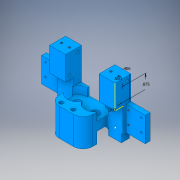
# Autodesk Inventor part: GripperBlock
Saved by Autodesk Inventor 2019 (Build 230136000, 136)
## iProperties
Created: 2019-10-02
Part Number: GripperBlock
Material: Generic
Document SubType Name: Modeling
Designer: james
Density: 1 g/cm^3
Appearance: Default(2)
Author: james
Autodesk Inventor part; units mm, degrees
ref_plane "YZ Plane" through (0, 0, 0) normal (1, 0, 0) x (0, 1, 0)
ref_plane "XZ Plane" through (0, 0, 0) normal (0, 1, 0) x (-1, 0, 0)
ref_plane "XY Plane" through (0, 0, 0) normal (0, 0, 1) x (1, 0, 0)
sketch "Sketch1" plane through (0, 0, 0) normal (1, 0, 0) x (0, 1, 0)
  line L0 (11.2985, 26.2091) -> (-33.1515, 26.2091)
  line L1 (-33.1515, 26.2091) -> (-33.1515, -24.5909)
  line L2 (-33.1515, -24.5909) -> (11.2985, -24.5909)
  line L3 (11.2985, -24.5909) -> (11.2985, 26.2091)
  point P0 (0, 0)
  dimension "d0" = 50.8
  dimension "d1" = 44.45
  constraints: 8 end point, 2 parallel, 1 horizontal, 1 perpendicular
  measures "d0" distance of L2.end L0.start
  measures "d1" distance of L0.start L0.end
extrude "Extrusion1" add sketch "Sketch1" along normal blind 165.1
sketch "Sketch2" plane through (0, 11.2985, 26.2091) normal (0, 1, 0) x (1, 0, 0)
  circle A0 centre (68.2625, 31.75) radius 15.875
  circle A1 centre (96.8375, 31.75) radius 15.875
  line L0 (0, 50.8) -> (0, 0) projected
  line L1 (0, 50.8) -> (165.1, 50.8) projected
  point P0 (0, 26.2091)
  dimension "d4" = 31.75
  dimension "d5" = 31.75
  dimension "d6" = 0
  dimension "d7" = 28.575
  dimension "d8" = 68.2625
  dimension "d9" = 19.05
  constraints: 2 centre point
  measures "d4" diameter of A0
  measures "d5" diameter of A1
  measures "d6" vertical distance of A0.centre A1.centre
  measures "d7" distance of A0.centre A1.centre
  measures "d8" distance from line of L0 A0.centre
  measures "d9" distance from line of L1 A0.centre
extrude "Extrusion2" cut sketch "Sketch2" against normal blind 12.7
sketch "Sketch3" plane through (0, -1.4015, 26.2091) normal (0, 1, 0) x (1, 0, 0)
  circle A0 centre (96.8375, 31.75) radius 15.875 projected
  circle A1 centre (68.2625, 31.75) radius 15.875 projected
  circle A2 centre (68.2625, 31.75) radius 3.302
  circle A3 centre (96.8375, 31.75) radius 3.302
  point P0 (0, 26.2091)
  point P1 (82.55, 38.6698)
  point P2 (82.55, 24.8302)
  dimension "d12" = 6.604
  dimension "d13" = 6.604
  constraints: 2 centre point, 2 coincident
  measures "d12" diameter of A2
  measures "d13" diameter of A3
extrude "Extrusion3" cut sketch "Sketch3" against normal blind 76.2 contours A2 | A3
sketch "Sketch4" plane through (0, -33.1515, -24.5909) normal (0, -1, 0) x (1, 0, 0)
  circle A0 centre (68.2625, 19.05) radius 3.302 projected
  circle A1 centre (96.8375, 19.05) radius 3.302 projected
  line L0 (0, 50.8) -> (0, 0) projected
  line L1 (0, 0) -> (165.1, 0) projected
  line L2 (165.1, 50.8) -> (165.1, 0) projected
  line L3 (0, 50.8) -> (165.1, 50.8) projected
  circle A2 centre (96.8375, 19.05) radius 3.302 projected
  circle A3 centre (68.2625, 19.05) radius 15.875
  circle A4 centre (96.8375, 19.05) radius 15.875
  point P0 (0, 24.5909)
  dimension "d16" = 31.75
  dimension "d17" = 31.75
  constraints: 2 centre point, 2 coincident
  measures "d16" diameter of A4
  measures "d17" diameter of A3
extrude "Extrusion4" cut sketch "Sketch4" against normal blind 17.78 contours A3 A4 | A3 A4 | A4 A3
sketch "Sketch5" plane through (0, -15.3715, -24.5909) normal (0, -1, 0) x (1, 0, 0)
  circle A0 centre (68.2625, 19.05) radius 3.302 projected
  circle A1 centre (96.8375, 19.05) radius 3.302 projected
  circle A2 centre (68.2625, 19.05) radius 6.35
  circle A3 centre (96.8375, 19.05) radius 6.35
  point P0 (0, 24.5909)
  dimension "d20" = 12.7
  dimension "d21" = 12.7
  constraints: 2 centre point, 2 coincident
  measures "d20" diameter of A2
  measures "d21" diameter of A3
extrude "Extrusion5" cut sketch "Sketch5" against normal blind 6.35
sketch "Sketch6" plane through (0, -1.4015, 26.2091) normal (0, 1, 0) x (1, 0, 0)
  circle A0 centre (68.2625, 31.75) radius 3.302 projected
  circle A1 centre (96.8375, 31.75) radius 3.302 projected
  circle A2 centre (68.2625, 31.75) radius 6.35
  circle A3 centre (96.8375, 31.75) radius 6.35
  point P0 (0, 26.2091)
  dimension "d24" = 12.7
  dimension "d25" = 12.7
  constraints: 2 centre point, 2 coincident
  measures "d24" diameter of A2
  measures "d25" diameter of A3
extrude "Extrusion6" cut sketch "Sketch6" against normal blind 6.35
sketch "Sketch7" plane through (0, -33.1515, -24.5909) normal (0, -1, 0) x (1, 0, 0)
  circle A0 centre (68.2625, 44.45) radius 3.175
  circle A1 centre (87.3125, 44.45) radius 3.175
  circle A2 centre (68.2625, 19.05) radius 3.302 projected
  circle A3 centre (96.8375, 19.05) radius 3.302 projected
  point P0 (0, 24.5909)
  dimension "d28" = 6.35
  dimension "d29" = 6.35
  dimension "d30" = 19.05
  dimension "d31" = 0
  dimension "d32" = 25.4
  dimension "d33" = 25.4
  constraints: 2 centre point
  measures "d28" diameter of A0
  measures "d29" diameter of A1
  measures "d30" distance of A0.centre A1.centre
  measures "d31" horizontal distance of A2.centre A0.centre
  measures "d32" distance of A0.centre A2.centre
  measures "d33" vertical distance of A3.centre A1.centre
extrude "Extrusion7" cut sketch "Sketch7" against normal blind 76.2 contours A0 | A1
sketch "Sketch8" plane through (0, 11.2985, 26.2091) normal (0, 1, 0) x (1, 0, 0)
  line L0 (-37.599, -14.8006) -> (55.88, -14.8006)
  line L1 (55.88, -14.8006) -> (55.88, 38.1)
  line L2 (55.88, 38.1) -> (-37.599, 38.1)
  line L3 (-37.599, 38.1) -> (-37.599, -14.8006)
  line L4 (109.22, -16.386) -> (193.9952, -16.386)
  line L5 (193.9952, -16.386) -> (193.9952, 38.1)
  line L6 (193.9952, 38.1) -> (109.22, 38.1)
  line L7 (109.22, 38.1) -> (109.22, -16.386)
  line L8 (0, 50.8) -> (165.1, 50.8) projected
  line L9 (0, 50.8) -> (0, 0) projected
  line L10 (165.1, 50.8) -> (165.1, 0) projected
  point P0 (0, 26.2091)
  dimension "d36" = 12.7
  dimension "d37" = 55.88
  dimension "d38" = 12.7
  dimension "d39" = 55.88
  constraints: 16 end point, 4 parallel, 2 horizontal, 2 perpendicular
  measures "d36" distance between parallel lines of L2 L8
  measures "d37" distance between parallel lines of L9 L1
  measures "d38" distance between parallel lines of L8 L6
  measures "d39" distance between parallel lines of L10 L7
extrude "Extrusion8" cut sketch "Sketch8" against normal blind 76.2
fillet "Fillet1" radius 15.24 1 edges at (109.22, -10.9265, 26.2091)
fillet "Fillet2" radius 15.24 1 edges at (55.88, -10.9265, 26.2091)
sketch "Sketch10" plane through (0, 11.2985, -24.5909) normal (0, 1, 0) x (1, 0, 0)
  circle A0 centre (68.2625, -19.05) radius 6.35 projected
  circle A1 centre (96.8375, -19.05) radius 6.35 projected
  line L0 (68.2625, -19.05) -> (96.8375, -19.05)
  line L1 (96.8375, -19.05) -> (96.8375, 8.338)
  line L2 (96.8375, 8.338) -> (68.2625, 8.338)
  line L3 (68.2625, 8.338) -> (68.2625, -19.05)
  point P0 (0, -24.5909)
  dimension "d46" = 0
  dimension "d47" = 0
  dimension "d48" = 0
  constraints: 8 end point, 2 parallel, 1 horizontal, 1 perpendicular
  measures "d46" distance from line of A1.centre L1
  measures "d47" distance from line of A1.centre L0
  measures "d48" distance from line of L3 A0.centre
extrude "Extrusion9" cut sketch "Sketch10" against normal blind 12.7 contours L0 L3 A0 | A0 L3 L2 L1 A1 L0 | A1 L1 L0 picked at (71.2371, -16.0754) picked at (95.4481, -15.0794)
sketch "Sketch11" plane through (0, 11.2985, -11.8909) normal (0, 1, 0) x (1, 0, 0)
  line L0 (165.1, 0) -> (109.22, 0)
  line L1 (109.22, 0) -> (109.22, 12.7)
  line L2 (109.22, 12.7) -> (165.1, 12.7)
  line L3 (165.1, 12.7) -> (165.1, 0)
  line L4 (55.88, 0) -> (0, 0)
  line L5 (0, 0) -> (0, 12.7)
  line L6 (0, 12.7) -> (55.88, 12.7)
  line L7 (55.88, 12.7) -> (55.88, 0)
  line L8 (109.22, -22.86) -> (109.22, -16.2842) projected
  line L9 (96.8375, 12.7) -> (165.1, 12.7) projected
  line L10 (111.3872, 0) -> (165.1, 0) projected
  line L11 (55.88, -16.2842) -> (55.88, -22.86) projected
  line L12 (0, 0) -> (53.7128, 0) projected
  line L13 (0, 12.7) -> (68.2625, 12.7) projected
  line L14 (0, 12.7) -> (0, 0) projected
  line L15 (165.1, 12.7) -> (165.1, 0) projected
  point P0 (0, -11.8909)
  point P1 (109.22, 0)
  point P2 (55.88, 0)
  dimension "d54" = 0
  dimension "d55" = 0
  dimension "d57" = 0
  dimension "d58" = 0
  dimension "d59" = 0
  dimension "d60" = 0
  dimension "d120" = 0
  dimension "d121" = 0
  dimension "d122" = 53.34
  constraints: 16 end point, 4 parallel, 2 horizontal, 2 perpendicular
  measures "d54" distance between parallel lines of L9 L2
  measures "d55" distance between parallel lines of L10 L0
  measures "d57" distance between parallel lines of L12 L4
  measures "d58" distance between parallel lines of L6 L13
  measures "d59" distance between parallel lines of L14 L5
  measures "d60" distance between parallel lines of L15 L3
  measures "d120" distance between parallel lines of L7 L11
  measures "d121" distance between parallel lines of L8 L1
  measures "d122" distance between parallel lines of L1 L7
extrude "Extrusion10" add sketch "Sketch11" along normal blind 12.7
sketch "Sketch12" plane through (0, 23.9985, -11.8909) normal (0, 1, 0) x (1, 0, 0)
  line L0 (134.62, -12.7) -> (109.22, -12.7)
  line L1 (109.22, -12.7) -> (109.22, 12.7)
  line L2 (109.22, 12.7) -> (134.62, 12.7)
  line L3 (134.62, 12.7) -> (134.62, -12.7)
  line L4 (55.88, -12.7) -> (30.48, -12.7)
  line L5 (30.48, -12.7) -> (30.48, 12.7)
  line L6 (30.48, 12.7) -> (55.88, 12.7)
  line L7 (55.88, 12.7) -> (55.88, -12.7)
  line L8 (165.1, 12.7) -> (109.22, 12.7) projected
  line L9 (55.88, 12.7) -> (0, 12.7) projected
  line L10 (55.88, -16.2842) -> (55.88, -22.86) projected
  line L11 (109.22, -22.86) -> (109.22, -16.2842) projected
  line L12 (55.88, 0) -> (55.88, 12.7) projected
  line L13 (109.22, 12.7) -> (109.22, 0) projected
  point P0 (0, -11.8909)
  point P1 (55.88, 0)
  dimension "d63" = 25.4
  dimension "d64" = 25.4
  dimension "d65" = 0
  dimension "d66" = 0
  dimension "d68" = 25.4
  dimension "d69" = 25.4
  dimension "d123" = 0
  dimension "d124" = 0
  constraints: 16 end point, 4 parallel, 2 horizontal, 2 perpendicular
  measures "d63" distance of L5.end L6.end
  measures "d64" distance of L1.end L2.end
  measures "d65" distance between parallel lines of L2 L8
  measures "d66" distance between parallel lines of L9 L6
  measures "d68" distance between parallel lines of L6 L4
  measures "d69" distance between parallel lines of L2 L0
  measures "d123" distance between parallel lines of L7 L12
  measures "d124" distance between parallel lines of L1 L13
extrude "Extrusion11" add sketch "Sketch12" along normal blind 38.1
sketch "Sketch13" plane through (134.62, 23.9985, 0.8091) normal (1, 0, 0) x (0, 0, -1)
  line L0 (0, 0) -> (0, 38.1) projected
  line L1 (12.7, 0) -> (0, 0) projected
  point P0 (0.8091, -23.9985)
  point P1 (6.35, 6.35)
  point P2 (19.05, 31.75)
  dimension "d73" = 6.35
  dimension "d74" = 6.35
  dimension "d75" = 31.75
  dimension "d76" = 19.05
  measures "d73" distance from line of point (6.35, 6.35) L0
  measures "d74" distance from line of L1 point (6.35, 6.35)
  measures "d75" distance from line of L1 point (19.05, 31.75)
  measures "d76" distance from line of L0 point (19.05, 31.75)
hole "Hole1" at (134.62, 30.3485, -5.5409) at (134.62, 55.7485, -18.2409) direction (-1, 0, 0) diameter 4.4958 end through all clearance for "Flat Head Machine Screw (82)" size "#8" standard "Ansi Unified Screw Threads"
sketch "Sketch17" plane through (0, 62.0985, -11.8909) normal (0, 1, 0) x (1, 0, 0)
  line L0 (134.62, 12.7) -> (109.22, 12.7) projected
  line L1 (134.62, -12.7) -> (134.62, 12.7) projected
  line L2 (109.22, 12.7) -> (109.22, -12.7) projected
  line L3 (30.48, 12.7) -> (30.48, -12.7) projected
  line L4 (55.88, -12.7) -> (55.88, 12.7) projected
  line L5 (55.88, 12.7) -> (30.48, 12.7) projected
  point P0 (0, -11.8909)
  point P1 (36.83, 0)
  point P2 (49.53, 0)
  point P3 (115.57, 0)
  point P4 (128.27, 0)
  dimension "d103" = 12.7
  dimension "d104" = 6.35
  dimension "d107" = 6.35
  dimension "d108" = 0
  dimension "d109" = 6.35
  dimension "d110" = 6.35
  dimension "d111" = 12.7
  dimension "d112" = 12.7
  measures "d103" distance from line of L0 point (128.27, 0)
  measures "d104" distance from line of L1 point (128.27, 0)
  measures "d107" distance from line of L2 point (115.57, 0)
  measures "d108" vertical distance of point (128.27, 0) point (115.57, 0)
  measures "d109" distance from line of L3 point (36.83, 0)
  measures "d110" distance from line of L4 point (49.53, 0)
  measures "d111" distance from line of L5 point (49.53, 0)
  measures "d112" distance from line of L5 point (36.83, 0)
hole "Hole2" at (36.83, 62.0985, -11.8909) at (49.53, 62.0985, -11.8909) at (115.57, 62.0985, -11.8909) at (128.27, 62.0985, -11.8909) direction (0, -1, 0) diameter 3.302 depth 25.4 tip angle 118.188 thread size "8-32 UNC" class "2B" standard "ANSI Unified Screw Threads"
sketch "Sketch18" plane through (165.1, 0, 0) normal (1, 0, 0) x (0, 0, -1)
  line L0 (11.8909, -28.0715) -> (34.8193, -28.0715)
  line L1 (34.8193, -28.0715) -> (34.8193, -40.9464)
  line L2 (34.8193, -40.9464) -> (11.8909, -40.9464)
  line L3 (11.8909, -40.9464) -> (11.8909, -28.0715)
  line L4 (11.8909, -33.1515) -> (24.5909, -33.1515) projected
  line L5 (11.8909, -33.1515) -> (11.8909, 23.9985) projected
  point P0 (0, 0)
  dimension "d125" = 5.08
  dimension "d126" = 0
  constraints: 8 end point, 2 parallel, 1 horizontal, 1 perpendicular
  measures "d125" distance between parallel lines of L4 L0
  measures "d126" distance between parallel lines of L5 L3
extrude "Extrusion14" cut sketch "Sketch18" against normal blind 185.7375
sketch "Sketch19" plane through (96.8375, -1.4015, -24.5909) normal (0, 0, -1) x (-1, 0, 0)
  line L0 (63.8175, -33.8983) -> (99.5096, -33.8983)
  line L1 (99.5096, -33.8983) -> (99.5096, -13.97)
  line L2 (99.5096, -13.97) -> (63.8175, -13.97)
  line L3 (63.8175, -13.97) -> (63.8175, -33.8983)
  line L4 (-35.2425, -40.1175) -> (-92.1403, -40.1175)
  line L5 (-92.1403, -40.1175) -> (-92.1403, -13.97)
  line L6 (-92.1403, -13.97) -> (-35.2425, -13.97)
  line L7 (-35.2425, -13.97) -> (-35.2425, -40.1175)
  line L8 (-68.2625, -26.67) -> (96.8375, -26.67) projected
  line L9 (-68.2625, -26.67) -> (-68.2625, 25.4) projected
  line L10 (96.8375, -26.67) -> (96.8375, 25.4) projected
  point P0 (96.8375, 1.4015)
  dimension "d129" = 12.7
  dimension "d130" = 33.02
  dimension "d131" = 33.02
  dimension "d132" = 12.7
  constraints: 16 end point, 4 parallel, 2 horizontal, 2 perpendicular
  measures "d129" distance between parallel lines of L8 L6
  measures "d130" distance between parallel lines of L9 L7
  measures "d131" distance between parallel lines of L10 L3
  measures "d132" distance between parallel lines of L8 L2
extrude "Extrusion17" cut sketch "Sketch19" against normal blind 185.7375
sketch "Sketch22" plane through (0, 23.9985, -11.8909) normal (0, 1, 0) x (1, 0, 0)
  line L0 (0, -16.8208) -> (30.48, -16.8208)
  line L1 (30.48, -16.8208) -> (30.48, 5.08)
  line L2 (30.48, 5.08) -> (0, 5.08)
  line L3 (0, 5.08) -> (0, -16.8208)
  line L4 (30.48, 12.7) -> (30.48, -12.7) projected
  line L5 (0, 12.7) -> (0, 0) projected
  line L6 (0, 0) -> (30.48, 0) projected
  point P0 (0, -11.8909)
  dimension "d140" = 0
  dimension "d141" = 0
  dimension "d142" = 5.08
  constraints: 8 end point, 2 parallel, 1 horizontal, 1 perpendicular
  measures "d140" distance between parallel lines of L4 L1
  measures "d141" distance between parallel lines of L5 L3
  measures "d142" distance between parallel lines of L6 L2
extrude "Extrusion18" cut sketch "Sketch22" against normal blind 185.7375
sketch "Sketch23" plane through (0, 23.9985, -11.8909) normal (0, 1, 0) x (1, 0, 0)
  line L0 (175.2279, 5.08) -> (134.62, 5.08)
  line L1 (134.62, 5.08) -> (134.62, -15.5442)
  line L2 (134.62, -15.5442) -> (175.2279, -15.5442)
  line L3 (175.2279, -15.5442) -> (175.2279, 5.08)
  line L4 (134.62, -12.7) -> (134.62, 12.7) projected
  line L5 (134.62, 0) -> (165.1, 0) projected
  point P0 (0, -11.8909)
  dimension "d145" = 0
  dimension "d146" = 5.08
  constraints: 8 end point, 2 parallel, 1 horizontal, 1 perpendicular
  measures "d145" distance between parallel lines of L4 L1
  measures "d146" distance between parallel lines of L0 L5
extrude "Extrusion19" cut sketch "Sketch23" against normal blind 185.7375
sketch "Sketch24" plane through (0, 23.9985, -16.9709) normal (0, 0, 1) x (1, 0, 0)
  line L0 (0, -39.37) -> (0, 0) projected
  line L1 (30.48, 0) -> (30.48, -39.37) projected
  line L2 (0, 0) -> (30.48, 0) projected
  line L3 (30.48, -39.37) -> (0, -39.37) projected
  point P0 (0, -23.9985)
  point P1 (26.67, -6.35)
  point P2 (26.67, -26.67)
  point P3 (6.35, -26.67)
  point P4 (6.35, -6.35)
  dimension "d149" = 6.35
  dimension "d150" = 3.81
  dimension "d151" = 3.81
  dimension "d152" = 0
  dimension "d153" = 0
  dimension "d154" = 0
  dimension "d155" = 6.35
  dimension "d156" = 12.7
  measures "d149" distance from line of L0 point (6.35, -6.35)
  measures "d150" distance from line of L1 point (26.67, -6.35)
  measures "d151" distance from line of L1 point (26.67, -26.67)
  measures "d152" horizontal distance of point (6.35, -6.35) point (6.35, -26.67)
  measures "d153" vertical distance of point (26.67, -26.67) point (6.35, -26.67)
  measures "d154" vertical distance of point (26.67, -6.35) point (6.35, -6.35)
  measures "d155" distance from line of L2 point (26.67, -6.35)
  measures "d156" distance from line of L3 point (6.35, -26.67)
hole "Hole3" at (26.67, 17.6485, -16.9709) at (26.67, -2.6715, -16.9709) at (6.35, -2.6715, -16.9709) at (6.35, 17.6485, -16.9709) direction (0, 0, -1) diameter 2.6416 depth 10.9728 tip angle 118.188 thread size "6-32 UNC" class "2B" standard "ANSI Unified Screw Threads"
sketch "Sketch25" plane through (134.62, 23.9985, -16.9709) normal (0, 0, 1) x (1, 0, 0)
  line L0 (30.48, 0) -> (30.48, -39.37) projected
  line L1 (0, 0) -> (30.48, 0) projected
  line L2 (30.48, -39.37) -> (0, -39.37) projected
  line L3 (0, -39.37) -> (0, 0) projected
  point P0 (-134.62, -23.9985)
  point P1 (24.13, -6.35)
  point P2 (24.13, -26.67)
  point P3 (3.81, -6.35)
  point P4 (3.81, -26.67)
  dimension "d164" = 6.35
  dimension "d165" = 6.35
  dimension "d166" = 0
  dimension "d167" = 12.7
  dimension "d168" = 0
  dimension "d169" = 0
  dimension "d170" = 3.81
  dimension "d171" = 3.81
  measures "d164" distance from line of L0 point (24.13, -6.35)
  measures "d165" distance from line of L1 point (24.13, -6.35)
  measures "d166" horizontal distance of point (24.13, -6.35) point (24.13, -26.67)
  measures "d167" distance from line of L2 point (24.13, -26.67)
  measures "d168" vertical distance of point (24.13, -26.67) point (3.81, -26.67)
  measures "d169" vertical distance of point (24.13, -6.35) point (3.81, -6.35)
  measures "d170" distance from line of L3 point (3.81, -6.35)
  measures "d171" distance from line of L3 point (3.81, -26.67)
hole "Hole4" at (158.75, 17.6485, -16.9709) at (158.75, -2.6715, -16.9709) at (138.43, 17.6485, -16.9709) at (138.43, -2.6715, -16.9709) direction (0, 0, -1) diameter 2.6416 depth 10.9728 tip angle 118.188 thread size "6-32 UNC" class "2B" standard "ANSI Unified Screw Threads"
sketch "Sketch26" plane through (134.62, 23.9985, -24.5909) normal (1, 0, 0) x (0, 0, -1)
  line L0 (-12.7, 0) -> (-25.4, 0) projected
  line L1 (-25.4, 0) -> (-25.4, 38.1) projected
  point P0 (-24.5909, -23.9985)
  point P1 (-2.3876, 5.08)
  point P2 (-12.7, 27.305)
  dimension "d181" = 5.08
  dimension "d182" = 12.7
  dimension "d190" = 10.3124
  dimension "d191" = 22.225
  measures "d181" distance from line of L0 point (-2.388, 5.08)
  measures "d182" distance from line of L1 point (-12.7, 27.305)
  measures "d190" horizontal distance of point (-2.388, 5.08) point (-12.7, 27.305)
  measures "d191" vertical distance of point (-2.388, 5.08) point (-12.7, 27.305)
hole "Hole5" at (134.62, 29.0785, -22.2033) at (134.62, 51.3035, -11.8909) direction (-1, 0, 0) diameter 1.7018 depth 6.6294 tip angle 118.188
sketch "Sketch27" plane through (109.22, -28.0715, -11.8909) normal (0, 0, -1) x (-1, 0, 0)
  line L0 (-8.2156, -33.6683) -> (55.7272, -33.6683)
  line L1 (55.7272, -33.6683) -> (55.7272, 0)
  line L2 (55.7272, 0) -> (-8.2156, 0)
  line L3 (-8.2156, 0) -> (-8.2156, -33.6683)
  line L4 (-22.86, 0) -> (76.2, 0) projected
  point P0 (109.22, 28.0715)
  dimension "d192" = 0
  constraints: 8 end point, 2 parallel, 1 horizontal, 1 perpendicular
  measures "d192" distance between parallel lines of L4 L2
extrude "Extrusion20" [suppressed]
sketch "Sketch28" plane through (71.12, -28.0715, 26.2091) normal (0, -1, 0) x (1, 0, 0)
  arc A0 (38.1, -28.928) -> (38.1, -34.572) centre (25.7175, -31.75) ccw projected
  arc A1 (-15.24, -34.572) -> (-15.24, -28.928) centre (-2.8575, -31.75) ccw projected
  line L0 (-38.1, -38.1) -> (-17.4072, -38.1) projected
  line L1 (-38.1, -38.1) -> (-38.1, -50.8) projected
  line L2 (40.2672, -38.1) -> (60.96, -38.1) projected
  line L3 (-38.1, -38.1) -> (-17.4072, -38.1) projected
  line L4 (-38.1, -38.1) -> (-38.1, -50.8) projected
  line L5 (60.96, -50.8) -> (-38.1, -50.8) projected
  line L6 (60.96, -50.8) -> (60.96, -38.1) projected
  line L7 (40.2672, -38.1) -> (60.96, -38.1) projected
  arc A2 (-17.4072, -38.1) -> (11.43, -38.6698) centre (-2.8575, -31.75) ccw projected
  arc A3 (11.43, -38.6698) -> (40.2672, -38.1) centre (25.7175, -31.75) ccw projected
  point P0 (-71.12, -26.2091)
  point P1 (11.43, -23.3497)
  point P2 (-15.24, -38.1)
  point P3 (38.1, -38.1)
  point P4 (11.43, -13.1897)
  point P5 (-25.4, -44.45)
  point P6 (48.26, -44.45)
  dimension "d195" = 6.35
  dimension "d196" = 12.7
  dimension "d197" = 12.7
  dimension "d198" = 6.35
  dimension "d199" = 0
  dimension "d200" = 10.16
  constraints: 2 other
  measures "d195" distance from line of L0 point (-25.4, -44.45)
  measures "d196" distance from line of L1 point (-25.4, -44.45)
  measures "d197" distance from line of L6 point (48.26, -44.45)
  measures "d198" distance from line of L5 point (48.26, -44.45)
  measures "d199" horizontal distance of point (11.43, -13.19) point (11.43, -23.35)
  measures "d200" distance of point (11.43, -23.35) point (11.43, -13.19)
hole "Hole6" at (45.72, -28.0715, -18.2409) at (82.55, -28.0715, 13.0194) at (119.38, -28.0715, -18.2409) direction (0, 1, 0) diameter 3.302 depth 25.4 tip angle 118.188 counterbore diameter 6.985 counterbore depth 6.35 thread size "8-32 UNC" class "2B" standard "ANSI Unified Screw Threads"
body "Solid1"
